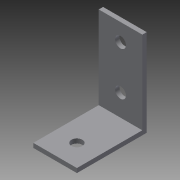
# Autodesk Inventor part: 000204
Saved by Autodesk Inventor 2015 (Build 190159000, 159)
## iProperties
Created: 2015-05-27
Part Number: 000204
Material: Generic
Document SubType Name: Modeling
Designer: Wesley
Density: 1 g/cm^3
Appearance: Default
Author: Wesley
Autodesk Inventor part; units mm, degrees
ref_plane "YZ Plane" through (0, 0, 0) normal (1, 0, 0) x (0, 1, 0)
ref_plane "XZ Plane" through (0, 0, 0) normal (0, 1, 0) x (-1, 0, 0)
ref_plane "XY Plane" through (0, 0, 0) normal (0, 0, 1) x (1, 0, 0)
sketch "Sketch1" plane through (0, 0, 0) normal (0, 0, 1) x (1, 0, 0)
  line L0 (0, 0) -> (12.7, 0)
  line L1 (12.7, 0) -> (12.7, 25.4)
  line L2 (12.7, 25.4) -> (0, 25.4)
  line L3 (0, 25.4) -> (0, 0)
  dimension "d0" = 25.4
  dimension "d1" = 12.7
  constraints: 8 end point, 2 parallel, 1 horizontal, 1 perpendicular
  measures "d0" distance of L2.end L0.start
  measures "d1" distance of L1.end L2.end
extrude "Extrusion1" add sketch "Sketch1" along normal blind 1.27
sketch "Sketch2" plane through (0, 0, 1.27) normal (0, 0, 1) x (1, 0, 0)
  line L0 (6.35, -14.9929) -> (6.35, 30.5291) construction
  line L1 (12.7, 0) -> (12.7, 25.4) construction
  line L2 (0, 0) -> (12.7, 0) projected
  point P0 (6.35, 20.32)
  point P1 (6.35, 7.62)
  dimension "d4" = 6.35
  dimension "d5" = 7.62
  dimension "d6" = 12.7
  constraints: 2 end point, 2 point on line, 1 vertical
  measures "d4" distance between parallel lines of L1 L0
  measures "d5" distance from line of L2 point (6.35, 7.62)
  measures "d6" distance of point (6.35, 20.32) point (6.35, 7.62)
hole "Hole1" at (6.35, 20.32, 1.27) at (6.35, 7.62, 1.27) direction (0, 0, -1) diameter 3.175 depth 25.4 tip angle 118
sketch "Sketch3" plane through (0, 0, 1.27) normal (0, 0, 1) x (1, 0, 0)
  line L0 (12.7, 0) -> (12.7, 25.4) projected
  line L1 (0, 0) -> (12.7, 0)
  line L2 (12.7, 0) -> (12.7, 1.27)
  line L3 (12.7, 1.27) -> (0, 1.27)
  line L4 (0, 1.27) -> (0, 0)
  dimension "d14" = 1.27
  constraints: 8 end point, 2 parallel, 1 horizontal, 1 perpendicular, 1 point on line
  measures "d14" distance between parallel lines of L1 L3
extrude "Extrusion2" add sketch "Sketch3" along normal blind 19.05
sketch "Sketch4" plane through (0, 0, 0) normal (0, -1, 0) x (1, 0, 0)
  line L0 (6.35, -12.0636) -> (6.35, 31.9717) construction
  line L1 (12.7, 0) -> (12.7, 20.32) construction
  circle A0 centre (6.35, 13.97) radius 1.5875
  line L2 (0, 20.32) -> (12.7, 20.32) construction
  point P0 (0, 0)
  dimension "d17" = 6.35
  dimension "d18" = 3.175
  dimension "d19" = 6.35
  constraints: 2 end point, 1 centre point, 1 point on line, 1 vertical
  measures "d17" distance between parallel lines of L1 L0
  measures "d18" diameter of A0
  measures "d19" distance from line of L2 A0.centre
extrude "Extrusion3" cut sketch "Sketch4" against normal blind 19.05
body "Solid1"
